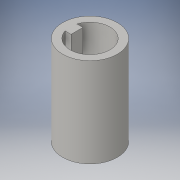
# Autodesk Inventor part: KeyedShaftCoupler
Saved by Autodesk Inventor 2016 (Build 200138000, 138)
## iProperties
Created: 2016-01-18
Part Number: KeyedShaftCoupler
Material: Generic
Document SubType Name: Modeling
Designer: yash
Density: 1 g/cm^3
Appearance: Default
Author: yash
Autodesk Inventor part; units mm, degrees
ref_plane "YZ Plane" through (0, 0, 0) normal (1, 0, 0) x (0, 1, 0)
ref_plane "XZ Plane" through (0, 0, 0) normal (0, 1, 0) x (-1, 0, 0)
ref_plane "XY Plane" through (0, 0, 0) normal (0, 0, 1) x (1, 0, 0)
sketch "Sketch1" plane through (0, 0, 0) normal (0, 1, 0) x (-1, 0, 0)
  circle A0 centre (0, 0) radius 11.6586
  arc A1 (8.0944, 2.54) -> (8.0944, -2.54) centre (0, 0) ccw
  line L0 (8.0944, 2.54) -> (5.5544, 2.54)
  line L1 (5.5544, 2.54) -> (5.5544, -2.54)
  line L2 (5.5544, -2.54) -> (8.0944, -2.54)
  point P0 (5.5544, 0)
  dimension "d0" = 23.3172
  dimension "d1" = 16.9672
  dimension "d3" = 5.08
  dimension "d4" = 2.54
  constraints: 6 end point, 2 centre point, 2 coincident, 2 point on circle, 1 horizontal, 1 horizontal alignment, 1 midpoint, 1 parallel, 1 perpendicular
  measures "d0" diameter of A0
  measures "d1" diameter of A1
  measures "d3" distance of L0.end L1.end
  measures "d4" distance of L1.end L2.end
extrude "Extrusion1" add sketch "Sketch1" along normal blind 38.1
body "Solid1"
